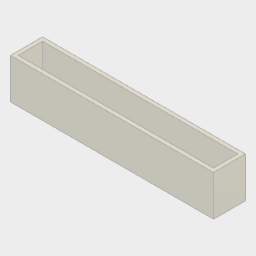
FingerOuterMold v3 (Autodesk Fusion 360 design; units mm, degrees)
Autodesk Fusion 360 part; units mm, degrees
sketch "Sketch1" plane through (0, 0, 0) normal (0, 1, 0) x (1, 0, 0)
  line L0 (0, 0) -> (105.6, 0)
  line L1 (105.6, 0) -> (105.6, 16.7)
  line L2 (105.6, 16.7) -> (0, 16.7)
  line L3 (0, 16.7) -> (0, 0)
  dimension "d1" = 105.6
  dimension "d2" = 16.7
  measures "d1" distance of L0.start L0.end
  measures "d2" distance of L0.start L2.end
extrude "Extrude1" add sketch "Sketch1" along normal blind 2
sketch "Sketch2" plane through (0, 2, 0) normal (0, 1, 0) x (-1, 0, 0)
  line L0 (0, -16.7) -> (0, 0)
  line L1 (0, 0) -> (-105.6, 0)
  line L2 (-105.6, 0) -> (-105.6, -16.7)
  line L3 (-105.6, -16.7) -> (0, -16.7)
  line L4 (0, 0) -> (-105.6, 0)
  line L5 (-105.6, 0) -> (-105.6, -16.7)
  line L6 (-105.6, -16.7) -> (0, -16.7)
  line L7 (0, -16.7) -> (0, 0)
  line L8 (-2, -2) -> (-103.6, -2)
  line L9 (-103.6, -2) -> (-103.6, -14.7)
  line L10 (-103.6, -14.7) -> (-2, -14.7)
  line L11 (-2, -14.7) -> (-2, -2)
  dimension "d5" = 2
extrude "Extrude2" add sketch "Sketch2" along normal blind 19.05
